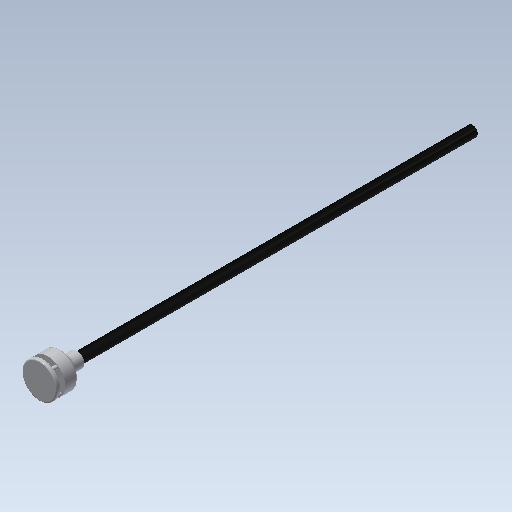
# Autodesk Inventor part: anemo
Saved by Autodesk Inventor 2020 (Build 240168000, 168)
## iProperties
Created: 2016-11-10
Part Number: anemo
Material: Generic
Document SubType Name: Modeling
Designer: jous
Density: 1 g/cm^3
Appearance: Default
Mass: 250.484 g
Surface Area: 512.39 cm^2
Volume: 250.484 cm^3
Author: jous
Autodesk Inventor part; units mm, degrees
ref_plane "YZ Plane" through (0, 0, 0) normal (1, 0, 0) x (0, 1, 0)
ref_plane "XZ Plane" through (0, 0, 0) normal (0, 1, 0) x (-1, 0, 0)
ref_plane "XY Plane" through (0, 0, 0) normal (0, 0, 1) x (1, 0, 0)
sketch "Sketch1" plane through (0, 0, 0) normal (0, 0, 1) x (1, 0, 0)
  circle A0 centre (0, 0) radius 9
  dimension "d0" = 18
  constraints: 1 centre point, 1 coincident
  measures "d0" diameter of A0
extrude "Extrusion1" add sketch "Sketch1" along normal blind 700
sketch "Sketch2" plane through (0, 0, 700) normal (0, 0, 1) x (1, 0, 0)
  circle A0 centre (0, 0) radius 9 projected
  circle A1 centre (0, 0) radius 30
  circle A2 centre (0, 0) radius 13
  dimension "d3" = 60
  dimension "d33" = 26
  constraints: 2 centre point, 2 coincident
  measures "d3" diameter of A1
  measures "d33" diameter of A2
extrude "Extrusion2" add sketch "Sketch2" along normal blind 30 contours A0 | A1 | A2
sketch "Sketch3" plane through (0, 0, 730) normal (0, 0, 1) x (1, 0, 0)
  circle A0 centre (0, 0) radius 30 projected
  line L0 (-24.495, 17.3203) -> (0, 0) construction
  line L1 (24.495, -17.3203) -> (0, 0) construction
  line L2 (0, 0) -> (17.3203, 24.495) construction
  line L3 (0, 0) -> (-17.3203, -24.495) construction
  circle A1 centre (-21.6666, 15.3203) radius 3
  circle A2 centre (-15.3203, -21.6666) radius 3
  circle A3 centre (21.6666, -15.3203) radius 3
  circle A4 centre (15.3203, 21.6666) radius 3
  dimension "d18" = 6
  dimension "d19" = 2
  dimension "d22" = 360
  constraints: 8 end point, 4 centre point, 4 point on circle, 2 collinear, 1 coincident, 1 perpendicular, 1 point on line, 9 other
  measures "d18" diameter of A1
  measures "d19" vertical distance of A1.centre L0.start
extrude "Extrusion3" add sketch "Sketch3" along normal blind 8.6 contours A1 | A2 | A3 | A4
sketch "Sketch4" plane through (0, 0, 738.6) normal (0, 0, 1) x (1, 0, 0)
  circle A0 centre (0, 0) radius 30
  dimension "d9" = 60
  constraints: 1 centre point, 1 coincident
  measures "d9" diameter of A0
extrude "Extrusion4" add sketch "Sketch4" along normal blind 6
chamfer "Chamfer2" distance 15.25 angle 30 1 edges at (-30, 0, 700) measured on face at (22.6222, -3.1111, 700)
fillet "Fillet5" radius 5 1 edges at (-30, 0, 708.8046)
extrude "Extrusion5" add sketch "Sketch2" against normal blind 20 contours A2
fillet "Fillet7" radius 20 1 edges at (-13, 0, 700)
fillet "Fillet8" radius 5 1 edges at (-14.75, 0, 700)
fillet "Fillet9" radius 2 1 edges at (-30, 0, 744.6)
body "Solid1"
